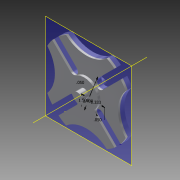
# Autodesk Inventor part: Geneva Driven
Saved by Autodesk Inventor 2018 (Build 220112000, 112)
## iProperties
Created: 2018-01-19
Part Number: Geneva Driven
Material: ABS Plastic
Document SubType Name: Modeling
Designer: Rus
Density: 1.06 g/cm^3
Appearance: Smooth - White
Mass: 106.579 g
Surface Area: 264.576 cm^2
Volume: 100.546 cm^3
Author: Rus
Autodesk Inventor part; units mm, degrees
ref_plane "YZ Plane" through (0, 0, 0) normal (1, 0, 0) x (0, 1, 0)
ref_plane "XZ Plane" through (0, 0, 0) normal (0, 1, 0) x (-1, 0, 0)
ref_plane "XY Plane" through (0, 0, 0) normal (0, 0, 1) x (1, 0, 0)
sketch "Sketch4" plane through (0, 0, 0) normal (0, 0, 1) x (1, 0, 0)
  line L0 (0, 0) -> (44.90085, -44.901711) construction
  line L1 (44.90085, -44.901711) -> (89.8017, 0) construction
  line L2 (89.8017, 0) -> (0, 0) construction
  circle A0 centre (0, 0) radius 63.5 construction
  line L3 (40.185611, -49.166724) -> (14.107761, -23.088374)
  line L4 (23.088103, -14.108204) -> (49.165953, -40.186554)
  arc A1 (23.088103, -14.108204) -> (14.107761, -23.088374) centre (18.597932, -18.598289) ccw
  arc A2 (56.350786, 29.27181) -> (56.350786, -29.27181) centre (89.8017, 0) ccw
  arc A3 (49.165953, -40.186554) -> (56.350786, -29.27181) centre (0, 0) ccw
  arc A4 (56.350786, 29.27181) -> (49.165953, 40.186554) centre (0, 0) ccw
  line L5 (49.165953, 40.186554) -> (56.350786, 29.27181) construction
  line L6 (56.350786, -29.27181) -> (49.165953, -40.186554) construction
  line L7 (0, 0) -> (44.901711, 44.90085) construction
  line L8 (44.901711, 44.90085) -> (0, 89.8017) construction
  line L9 (0, 89.8017) -> (0, 0) construction
  circle A5 centre (0, 0) radius 63.5 construction
  line L10 (49.165953, 40.186554) -> (23.088374, 14.107761)
  line L11 (14.108204, 23.088103) -> (40.186554, 49.165953)
  arc A6 (14.108204, 23.088103) -> (23.088374, 14.107761) centre (18.598289, 18.597932) ccw
  arc A7 (-29.27181, 56.350786) -> (29.27181, 56.350786) centre (0, 89.8017) ccw
  arc A8 (40.186554, 49.165953) -> (29.27181, 56.350786) centre (0, 0) ccw
  arc A9 (-29.27181, 56.350786) -> (-40.185611, 49.166724) centre (0, 0) ccw
  line L12 (-40.185611, 49.166724) -> (-29.27181, 56.350786) construction
  line L13 (29.27181, 56.350786) -> (40.186554, 49.165953) construction
  line L14 (0, 0) -> (-44.90085, 44.901711) construction
  line L15 (-44.90085, 44.901711) -> (-89.8017, 0) construction
  line L16 (-89.8017, 0) -> (0, 0) construction
  circle A10 centre (0, 0) radius 63.5 construction
  line L17 (-40.185611, 49.166724) -> (-14.107761, 23.088374)
  line L18 (-23.088103, 14.108204) -> (-49.165953, 40.186554)
  arc A11 (-23.088103, 14.108204) -> (-14.107761, 23.088374) centre (-18.597932, 18.598289) ccw
  arc A12 (-56.350786, -29.27181) -> (-56.350786, 29.27181) centre (-89.8017, 0) ccw
  arc A13 (-49.165953, 40.186554) -> (-56.350786, 29.27181) centre (0, 0) ccw
  arc A14 (-56.350786, -29.27181) -> (-49.166724, -40.185611) centre (0, 0) ccw
  line L19 (-49.166724, -40.185611) -> (-56.350786, -29.27181) construction
  line L20 (-56.350786, 29.27181) -> (-49.165953, 40.186554) construction
  line L21 (0, 0) -> (-44.901711, -44.90085) construction
  line L22 (-44.901711, -44.90085) -> (0, -89.8017) construction
  line L23 (0, -89.8017) -> (0, 0) construction
  circle A15 centre (0, 0) radius 63.5 construction
  line L24 (-49.166724, -40.185611) -> (-23.088374, -14.107761)
  line L25 (-14.108204, -23.088103) -> (-40.186554, -49.165953)
  arc A16 (-14.108204, -23.088103) -> (-23.088374, -14.107761) centre (-18.598289, -18.597932) ccw
  arc A17 (29.27181, -56.350786) -> (-29.27181, -56.350786) centre (0, -89.8017) ccw
  arc A18 (-40.186554, -49.165953) -> (-29.27181, -56.350786) centre (0, 0) ccw
  arc A19 (29.27181, -56.350786) -> (40.185611, -49.166724) centre (0, 0) ccw
  line L26 (40.185611, -49.166724) -> (29.27181, -56.350786) construction
  line L27 (-29.27181, -56.350786) -> (-40.186554, -49.165953) construction
  dimension "d22" = 89.8017
  dimension "d23" = 63.5
  dimension "d27" = 12.7
  dimension "d28" = 37.1983
  dimension "d29" = 44.45
  constraints: 56 end point, 56 point on circle, 20 centre point, 16 coincident, 4 point on line, 2 equal length, 2 parallel, 2 tangent, 1 concentric, 1 horizontal
  measures "d22" distance of L1.end L0.start
  measures "d23" distance of L0.end L1.end
  measures "d27" distance between parallel lines of L3 L4
  measures "d28" distance of A1.centre L0.end
  measures "d29" radius of A2
sketch "Sketch4 outline for Extrusion3" plane through (0, 0, 0) normal (0, 0, 1) x (1, 0, 0)
  arc A0 (29.27181, -56.350786) -> (40.185611, -49.166724) centre (0, 0) ccw
  arc A1 (-29.27181, -56.350786) -> (29.27181, -56.350786) centre (0, -89.8017) cw
  arc A2 (-40.186554, -49.165953) -> (-29.27181, -56.350786) centre (0, 0) ccw
  line L0 (-14.108204, -23.088103) -> (-40.186554, -49.165953)
  arc A3 (-23.088374, -14.107761) -> (-14.108204, -23.088103) centre (-18.598289, -18.597932) cw
  line L1 (-49.166724, -40.185611) -> (-23.088374, -14.107761)
  arc A4 (-56.350786, -29.27181) -> (-49.166724, -40.185611) centre (0, 0) ccw
  arc A5 (-56.350786, 29.27181) -> (-56.350786, -29.27181) centre (-89.8017, 0) cw
  arc A6 (-49.165953, 40.186554) -> (-56.350786, 29.27181) centre (0, 0) ccw
  line L2 (-23.088103, 14.108204) -> (-49.165953, 40.186554)
  arc A7 (-14.107761, 23.088374) -> (-23.088103, 14.108204) centre (-18.597932, 18.598289) cw
  line L3 (-40.185611, 49.166724) -> (-14.107761, 23.088374)
  arc A8 (-29.27181, 56.350786) -> (-40.185611, 49.166724) centre (0, 0) ccw
  arc A9 (29.27181, 56.350786) -> (-29.27181, 56.350786) centre (0, 89.8017) cw
  arc A10 (40.186554, 49.165953) -> (29.27181, 56.350786) centre (0, 0) ccw
  line L4 (14.108204, 23.088103) -> (40.186554, 49.165953)
  arc A11 (23.088374, 14.107761) -> (14.108204, 23.088103) centre (18.598289, 18.597932) cw
  line L5 (49.165953, 40.186554) -> (23.088374, 14.107761)
  arc A12 (56.350786, 29.27181) -> (49.165953, 40.186554) centre (0, 0) ccw
  arc A13 (56.350786, -29.27181) -> (56.350786, 29.27181) centre (89.8017, 0) cw
  arc A14 (49.165953, -40.186554) -> (56.350786, -29.27181) centre (0, 0) ccw
  line L6 (23.088103, -14.108204) -> (49.165953, -40.186554)
  arc A15 (14.107761, -23.088374) -> (23.088103, -14.108204) centre (18.597932, -18.598289) cw
  line L7 (40.185611, -49.166724) -> (14.107761, -23.088374)
extrude "Extrusion3" add sketch "Sketch4 outline for Extrusion3" along normal blind 16.933333
ref_plane "Work Plane1" through (0, 0, 8.466667) normal (0, 0, -1) x (-1, 0, 0)
sketch "Sketch13" plane through (0, 0, 0) normal (0, 0, -1) x (-1, 0, 0)
  circle A0 centre (0, 0) radius 11
  dimension "d68" = 22
  constraints: 1 centre point, 1 coincident
  measures "d68" diameter of A0
sketch "Sketch13 outline for Extrusion10" plane through (0, 0, 0) normal (0, 0, -1) x (-1, 0, 0)
  circle A0 centre (0, 0) radius 11
extrude "Extrusion10" cut sketch "Sketch13 outline for Extrusion10" against normal blind 7
sketch "Sketch14" plane through (0, 0, 16.933333) normal (0, 0, 1) x (1, 0, 0)
  circle A0 centre (0, 0) radius 11
  dimension "d71" = 22
  constraints: 1 centre point, 1 coincident
  measures "d71" diameter of A0
sketch "Sketch14 outline for Extrusion11" plane through (0, 0, 16.933333) normal (0, 0, 1) x (1, 0, 0)
  circle A0 centre (0, 0) radius 11
extrude "Extrusion11" cut sketch "Sketch14 outline for Extrusion11" against normal blind 7
sketch "Sketch15" plane through (0, 0, 9.933333) normal (0, 0, 1) x (1, 0, 0)
  circle A0 centre (0, 0) radius 11
  line L0 (40.185611, -49.166724) -> (14.107761, -23.088374)
  arc A1 (23.088103, -14.108204) -> (14.107761, -23.088374) centre (18.597932, -18.598289) ccw
  line L1 (23.088103, -14.108204) -> (49.165953, -40.186554)
  arc A2 (49.165953, -40.186554) -> (56.350786, -29.27181) centre (0, 0) ccw
  arc A3 (56.350786, 29.27181) -> (56.350786, -29.27181) centre (89.8017, 0) ccw
  arc A4 (56.350786, 29.27181) -> (49.165953, 40.186554) centre (0, 0) ccw
  line L2 (49.165953, 40.186554) -> (23.088374, 14.107761)
  arc A5 (14.108204, 23.088103) -> (23.088374, 14.107761) centre (18.598289, 18.597932) ccw
  line L3 (14.108204, 23.088103) -> (40.186554, 49.165953)
  arc A6 (40.186554, 49.165953) -> (29.27181, 56.350786) centre (0, 0) ccw
  arc A7 (-29.27181, 56.350786) -> (29.27181, 56.350786) centre (0, 89.8017) ccw
  arc A8 (-29.27181, 56.350786) -> (-40.185611, 49.166724) centre (0, 0) ccw
  line L4 (-40.185611, 49.166724) -> (-14.107761, 23.088374)
  arc A9 (-23.088103, 14.108204) -> (-14.107761, 23.088374) centre (-18.597932, 18.598289) ccw
  line L5 (-23.088103, 14.108204) -> (-49.165953, 40.186554)
  arc A10 (-49.165953, 40.186554) -> (-56.350786, 29.27181) centre (0, 0) ccw
  arc A11 (-56.350786, -29.27181) -> (-56.350786, 29.27181) centre (-89.8017, 0) ccw
  arc A12 (-56.350786, -29.27181) -> (-49.166724, -40.185611) centre (0, 0) ccw
  line L6 (-49.166724, -40.185611) -> (-23.088374, -14.107761)
  arc A13 (-14.108204, -23.088103) -> (-23.088374, -14.107761) centre (-18.598289, -18.597932) ccw
  line L7 (-14.108204, -23.088103) -> (-40.186554, -49.165953)
  arc A14 (-40.186554, -49.165953) -> (-29.27181, -56.350786) centre (0, 0) ccw
  arc A15 (29.27181, -56.350786) -> (-29.27181, -56.350786) centre (0, -89.8017) ccw
  arc A16 (29.27181, -56.350786) -> (40.185611, -49.166724) centre (0, 0) ccw
  circle A17 centre (0, 0) radius 3.175
  line L8 (-2.685749, -1.693333) -> (-10.868883, -1.693333)
  line L9 (-2.685749, 1.693333) -> (-10.868883, 1.693333)
  line L10 (-1.693333, 2.685749) -> (-1.693333, 10.868883)
  line L11 (1.693333, 2.685749) -> (1.693333, 10.868883)
  line L12 (1.693333, -2.685749) -> (1.693333, -10.868883)
  line L13 (-1.693333, -2.685749) -> (-1.693333, -10.868883)
  line L14 (2.685749, -1.693333) -> (10.868883, -1.693333)
  line L15 (2.685749, 1.693333) -> (10.868883, 1.693333)
  circle A18 centre (0, 0) radius 10.25
  line L16 (-6.777316, 1.693333) -> (-6.777316, -1.693333) construction
  line L17 (-1.693333, 6.777316) -> (1.693333, 6.777316) construction
  line L18 (6.777316, 1.693333) -> (6.777316, -1.693333) construction
  line L19 (-1.693333, -6.777316) -> (1.693333, -6.777316) construction
  point P0 (-6.777316, 0)
  dimension "d74" = 6.35
  dimension "d75" = 0.75
  dimension "d76" = 3.38667
  constraints: 24 end point, 9 midpoint, 5 horizontal, 5 vertical, 3 perpendicular, 2 coincident, 2 parallel, 1 centre point, 19 other
  measures "d76" distance between parallel lines of L9 L8
sketch "Sketch15 outline for Extrusion12" plane through (0, 0, 9.933333) normal (0, 0, 1) x (1, 0, 0)
  arc A0 (-1.693333, -2.685749) -> (-2.685749, -1.693333) centre (0, 0) cw
  line L0 (-1.693333, -10.868883) -> (-1.693333, -2.685749)
  arc A1 (-10.868883, -1.693333) -> (-1.693333, -10.868883) centre (0, 0) ccw
  line L1 (-2.685749, -1.693333) -> (-10.868883, -1.693333)
  line L2 (-10.868883, 1.693333) -> (-2.685749, 1.693333)
  arc A2 (-1.693333, 10.868883) -> (-10.868883, 1.693333) centre (0, 0) ccw
  line L3 (-1.693333, 2.685749) -> (-1.693333, 10.868883)
  arc A3 (-2.685749, 1.693333) -> (-1.693333, 2.685749) centre (0, 0) cw
  line L4 (1.693333, 10.868883) -> (1.693333, 2.685749)
  arc A4 (10.868883, 1.693333) -> (1.693333, 10.868883) centre (0, 0) ccw
  line L5 (2.685749, 1.693333) -> (10.868883, 1.693333)
  arc A5 (1.693333, 2.685749) -> (2.685749, 1.693333) centre (0, 0) cw
  arc A6 (2.685749, -1.693333) -> (1.693333, -2.685749) centre (0, 0) cw
  line L6 (10.868883, -1.693333) -> (2.685749, -1.693333)
  arc A7 (1.693333, -10.868883) -> (10.868883, -1.693333) centre (0, 0) ccw
  line L7 (1.693333, -2.685749) -> (1.693333, -10.868883)
extrude "Extrusion12" cut sketch "Sketch15 outline for Extrusion12" against normal blind 7
ref_plane "Work Plane4" through (-10.868883, 0, 9.933333) normal (0, -1, 0) x (1, 0, 0)
sketch "Sketch16" plane through (-10.868883, 0, 9.933333) normal (0, -1, 0) x (1, 0, 0)
  line L0 (-0.131117, 7) -> (-0.131117, -9.933333)
  line L1 (-0.131117, 0.25) -> (0.118883, 0.25) construction
  line L2 (0.118883, 0.25) -> (0.118883, 0) construction
  line L3 (0.118883, -3.183333) -> (-0.131117, -3.183333) construction
  line L4 (-0.131117, -1.466667) -> (0.118883, -1.466667)
  line L5 (8.183134, -2.933333) -> (0, -2.933333)
  line L6 (0.118883, -2.933333) -> (-0.131117, -3.183333)
  line L7 (0, 0) -> (8.183134, 0)
  line L8 (0.118883, 0) -> (-0.131117, 0.25)
  line L9 (0.118883, 0) -> (0.118883, -2.933333)
  line L10 (0.118883, -2.933333) -> (0.118883, -3.183333) construction
  line L11 (21.868883, -9.933333) -> (-0.131117, -9.933333)
  line L12 (-0.131117, 7) -> (21.868883, 7)
  line L13 (10.868883, -9.933333) -> (10.868883, 7) construction
  dimension "d79" = 0.25
  dimension "d80" = 0.25
  constraints: 18 end point, 8 perpendicular, 5 point on line, 2 midpoint, 1 horizontal
  measures "d79" distance between parallel lines of L2 L0
  measures "d80" distance between parallel lines of L3 L5
sketch "Sketch16 outline for Revolution2" plane through (-10.868883, 0, 9.933333) normal (0, -1, 0) x (1, 0, 0)
  line L0 (0.118883, 0) -> (-0.131117, 0.25)
  line L1 (0.118883, -2.933333) -> (0.118883, 0)
  line L2 (-0.131117, -3.183333) -> (0.118883, -2.933333)
  line L3 (-0.131117, -1.466667) -> (-0.131117, -3.183333)
  line L4 (-0.131117, 0.25) -> (-0.131117, -1.466667)
revolve "Revolution2" add sketch "Sketch16 outline for Revolution2" angle 360 about axis through (0, 0, 0) along (0, 0, 1)
sketch "Sketch17" plane through (0, 0, 9.933333) normal (0, 0, 1) x (1, 0, 0)
  circle A0 centre (0, 0) radius 5
  dimension "d82" = 10
  constraints: 1 centre point, 1 coincident
  measures "d82" diameter of A0
sketch "Sketch17 outline for Extrusion13" plane through (0, 0, 9.933333) normal (0, 0, 1) x (1, 0, 0)
  circle A0 centre (0, 0) radius 5
extrude "Extrusion13" cut sketch "Sketch17 outline for Extrusion13" against normal up to surface (2.933333 mm away)
sketch "Sketch18" plane through (0, 0, 9.933333) normal (0, 0, 1) x (1, 0, 0)
  arc A0 (-1.693333, -4.704532) -> (1.693333, -4.704532) centre (0, 0) ccw
  circle A1 centre (0, 0) radius 5
  circle A2 centre (0, 0) radius 6.5
  circle A3 centre (0, 0) radius 11
  arc A4 (10.615796, 1.693333) -> (1.693333, 10.615796) centre (0, 0) ccw
  line L0 (0, 0) -> (11, 0) construction
  dimension "d85" = 1.5
  constraints: 2 coincident, 2 end point, 1 centre point, 1 horizontal, 3 other
sketch "Sketch18 outline for Extrusion14" plane through (0, 0, 9.933333) normal (0, 0, 1) x (1, 0, 0)
  circle A0 centre (0, 0) radius 6.5
  circle A1 centre (0, 0) radius 5
extrude "Extrusion14" add sketch "Sketch18 outline for Extrusion14" against normal up to surface (2.933333 mm away)
body "Solid2"
